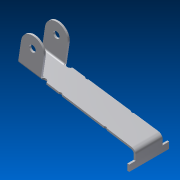
# Autodesk Inventor part: Omron SS-01GL2-E Microswitch Spring Lever
Saved by Autodesk Inventor 2013 (Build 170138000, 138)
## iProperties
Created: 2012-05-23
Part Number: Omron SS-01GL2-E Microswitch Spring Lever
Material: Stainless Steel
Document SubType Name: Modeling
Designer: sdarley
Density: 1 g/cm^3
Author: sdarley
Autodesk Inventor part; units mm, degrees
ref_plane "YZ Plane" through (0, 0, 0) normal (1, 0, 0) x (0, 1, 0)
ref_plane "XZ Plane" through (0, 0, 0) normal (0, 1, 0) x (-1, 0, 0)
ref_plane "XY Plane" through (0, 0, 0) normal (0, 0, 1) x (1, 0, 0)
sketch "Sketch1" plane through (0, 0, 0) normal (0, 1, 0) x (-1, 0, 0)
  line L0 (-0.15, 0) -> (0.15, 0)
  line L1 (0.15, 0) -> (0.15, 1.8)
  line L2 (-0.15, 0) -> (-0.15, 1.8)
  line L3 (0.553963, 2.268822) -> (18.4, 4.93593)
  line L4 (18.4, 4.93593) -> (18.355657, 5.232635)
  line L5 (18.355657, 5.232635) -> (0.50962, 2.565526)
  arc A0 (0.553963, 2.268822) -> (0.15, 1.8) centre (0.624029, 1.8) ccw
  arc A1 (0.50962, 2.565526) -> (-0.15, 1.8) centre (0.624029, 1.8) ccw
  point P0 (0, 0)
  point P1 (0, 0)
  dimension "d0" = 0.3
  dimension "d1" = 0.3
  dimension "d2" = 0.3
  dimension "d3" = 1.8
  dimension "d4" = 0.40396
  dimension "d5" = 8.5
  dimension "d6" = 18.55
  constraints: 12 end point, 5 point on circle, 4 tangent, 2 centre point, 2 coincident, 2 parallel, 2 perpendicular, 1 horizontal, 1 midpoint, 1 point on line
  measures "d0" distance of L0.start L0.end
  measures "d1" distance of L3.end L4.end
  measures "d2" radial gap between concentric circles of A1 A0
  measures "d3" distance of L0.start L2.end
  measures "d4" distance from line of L3 L1.end
  measures "d5" angle of L0 L3
  measures "d6" distance from line of L3.end L2
extrude "Extrusion1" add sketch "Sketch1" along normal mid plane 4.25
sketch "Sketch2" plane through (-0.15, -2.125, 1.8) normal (-1, 0, 0) x (0, 0, 1)
  line L0 (-1.8, 4.25) -> (-0.8, 4.25)
  line L1 (-0.8, 4.25) -> (-0.8, 5.25)
  line L2 (-0.8, 5.25) -> (-1.8, 5.25)
  line L3 (-1.8, 5.25) -> (-1.8, 4.25)
  line L4 (-1.8, 0) -> (-0.8, 0)
  line L5 (-0.8, 0) -> (-0.8, -1)
  line L6 (-0.8, -1) -> (-1.8, -1)
  line L7 (-1.8, -1) -> (-1.8, 0)
  point P0 (-1.8, 2.125)
  dimension "d9" = 1
  dimension "d10" = 1
  dimension "d11" = 1
  dimension "d12" = 1
  constraints: 16 end point, 4 parallel, 2 horizontal, 2 perpendicular
  measures "d9" distance of L2.end L1.end
  measures "d10" distance of L1.end L0.end
  measures "d11" distance of L5.end L6.end
  measures "d12" distance of L4.end L5.end
extrude "Extrusion2" add sketch "Sketch2" against normal up to surface (0.3 mm away)
sketch "Sketch3" plane through (-0.50962, -2.125, 2.565526) normal (0.1478094, 0, 0.9890159) x (0.9890159, 0, -0.1478094)
  line L0 (-18.044238, 4.25) -> (0, 4.25)
  line L1 (-18.044238, 0) -> (-18.044238, 4.25)
  line L2 (0, 0) -> (-18.044238, 0)
  line L3 (-18.044238, 4.15) -> (-18.044238, 0.1)
  line L4 (0, 0) -> (0, 4.25)
  line L5 (-18.044238, 2.125) -> (0, 2.125) construction
  arc A0 (-11.516226, 4.170271) -> (-11.016226, 4.173733) centre (-11.267189, 4.311097) ccw
  line L6 (0.883774, 4.25) -> (0.883774, 5.25)
  arc A1 (-4.366226, 4.219772) -> (-3.866226, 4.223233) centre (-4.117586, 4.417967) ccw
  arc A2 (-11.016226, 0.076267) -> (-11.516226, 0.079729) centre (-11.267189, -0.061097) ccw
  arc A3 (-3.866226, 0.026767) -> (-4.366226, 0.030228) centre (-4.117586, -0.167967) ccw
  line L7 (-18.044238, 4.15) -> (-14.444238, 4.15)
  line L8 (-14.444238, 4.15) -> (0, 4.25)
  line L9 (-14.444238, 0.1) -> (0, 0)
  line L10 (-18.044238, 0.1) -> (-14.444238, 0.1)
  arc A4 (-18.044238, 1.05) -> (-18.044238, 3.2) centre (-18.949863, 2.125) ccw
  arc A5 (-14.444238, 4.15) -> (-13.544238, 4.156231) centre (-13.994581, 4.202739) ccw
  arc A6 (-13.544238, 0.093769) -> (-14.444238, 0.1) centre (-13.994581, 0.047261) ccw
  point P0 (0.883231, 2.125)
  dimension "d15" = 4.05
  dimension "d19" = 0.5
  dimension "d20" = 1.9
  dimension "d21" = 11.9
  dimension "d22" = 0.5
  dimension "d23" = 1.975
  dimension "d24" = 4.75
  dimension "d25" = 1.9
  dimension "d26" = 1.975
  dimension "d27" = 3.6
  dimension "d28" = 2.15
  dimension "d29" = 0.5
  dimension "d35" = 1.625
  dimension "d36" = 0.9
  dimension "d37" = 1.625
  constraints: 14 point on circle, 14 point on line, 12 end point, 7 centre point, 6 vertical alignment, 4 midpoint, 2 perpendicular, 1 coincident, 1 horizontal alignment, 1 parallel
  measures "d15" distance of L3.end L3.start
  measures "d19" distance of A0.end A0.start
  measures "d20" distance edge to line of A0 L5
  measures "d21" distance from line of A0.end L6
  measures "d22" distance of A1.end A1.start
  measures "d23" distance edge to line of A1 L5
  measures "d24" distance from line of A1.end L6
  measures "d25" distance edge to line of A2 L5
  measures "d26" distance edge to line of A3 L5
  measures "d27" distance of L3.start L7.end
  measures "d28" distance of A4.start A4.end
  measures "d29" distance edge to line of A4 L3
  measures "d35" distance edge to line of A5 L5
  measures "d36" horizontal distance of A5.end L7.end
  measures "d37" distance edge to line of A6 L5
extrude "Extrusion3" cut sketch "Sketch3" against normal through all contours L0 L8 L7 L1 | L2 L1 L10 L9 | A1 L8 | A4 L1 | L8 A5 | L9 A3 | A0 L8 | A6 L9 | L9 A2
sketch "Sketch4" plane through (-18.355657, 2.025, 5.232635) normal (0, 1, 0) x (0.9890159, 0, -0.1478094)
  line L0 (0, 0.3) -> (3.6, 0.3)
  line L1 (3.6, 0) -> (0, 0)
  line L2 (3.6, 0) -> (3.6, 0.3)
  line L3 (3.6, 0) -> (3.6, -3.1)
  line L4 (0, 0) -> (0, -3.1)
  arc A0 (0, -3.1) -> (3.6, -3.1) centre (1.8, -3.1) ccw
  circle A1 centre (1.8, -3.1) radius 0.5
  point P0 (18.927469, 2.46202)
  point P1 (1.8, 0)
  dimension "d30" = 5.2
  dimension "d31" = 1
  constraints: 10 end point, 2 centre point, 2 point on circle, 1 coincident, 1 collinear, 1 midpoint, 1 parallel, 1 tangent, 1 vertical alignment
  measures "d31" diameter of A1
extrude "Extrusion4" add sketch "Sketch4" against normal blind 0.3
mirror "Mirror1" about plane through (0, 0, 0) normal (0, 1, 0) of "Extrusion4"
fillet "Fillet1" radius 0.25 2 edges at (-16.5754, 1.725, 4.9666) (-16.5754, -1.725, 4.9666)
fillet "Fillet2" radius 0.4 2 edges at (-16.6198, 2.025, 4.6699) (-16.6198, -2.025, 4.6699)
equation "\"d1\" = d0"
equation "\"d2\" = d0"
equation "\"d22\" = d19"
equation "\"d25\" = d20"
equation "\"d26\" = d23"
equation "\"d37\" = d35"
body "Solid1"
